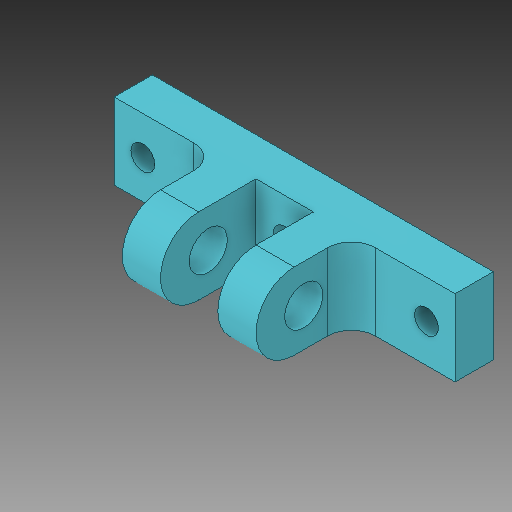
# Autodesk Inventor part: LowerSpringMountFront
Saved by Autodesk Inventor 2018.2 (Build 222227000, 227)
## iProperties
Created: 2018-03-25
Part Number: LowerSpringMountFront
Material: Generic
Document SubType Name: Modeling
Designer: MIABo
Density: 1 g/cm^3
Appearance: Default
Mass: 3.25903 g
Surface Area: 23.365 cm^2
Volume: 3.25903 cm^3
Author: MIABo
## iProperties of the stored document LowerSpringMountFront_3DPrint.ipt
Created: 2018-03-25
Part Number: LowerSpringMountFront_3DPrint
Material: Generic
Document SubType Name: Modeling
Designer: MIABo
Density: 1 g/cm^3
Appearance: Default
Author: MIABo
Autodesk Inventor part; units mm, degrees
ref_plane "YZ Plane" through (0, 0, 0) normal (1, 0, 0) x (0, 1, 0)
ref_plane "XZ Plane" through (0, 0, 0) normal (0, 1, 0) x (-1, 0, 0)
ref_plane "XY Plane" through (0, 0, 0) normal (0, 0, 1) x (1, 0, 0)
sketch "Sketch1" plane through (0, 0, 0) normal (0, 0, 1) x (1, 0, 0)
  line L0 (-22.6695, -5.08) -> (22.6695, -5.08)
  line L1 (22.6695, -5.08) -> (22.6695, 5.08)
  line L2 (22.6695, 5.08) -> (-22.6695, 5.08)
  line L3 (-22.6695, 5.08) -> (-22.6695, -5.08)
  line L4 (-22.6695, -5.08) -> (22.6695, 5.08) construction
  line L5 (22.6695, -5.08) -> (-22.6695, 5.08) construction
  point P0 (0, 0)
  dimension "d0" = 10.16
  dimension "d1" = 45.339
  constraints: 12 end point, 2 midpoint, 2 parallel, 1 horizontal, 1 perpendicular
  measures "d0" distance of L1.end L0.end
  measures "d1" distance of L1.end L2.end
extrude "Extrusion1" add sketch "Sketch1" along normal blind 5.08
sketch "Sketch2" plane through (0, 0, 0) normal (0, 0, -1) x (-1, 0, 0)
  line L0 (22.6695, 5.08) -> (22.6695, -5.08) projected
  line L1 (-22.6695, -5.08) -> (-22.6695, 5.08) projected
  line L2 (-22.6695, 5.08) -> (22.6695, 5.08) projected
  point P0 (0, 0)
  point P1 (18.8595, 0)
  point P2 (-18.8595, 0)
  dimension "d4" = 3.81
  dimension "d5" = 3.81
  dimension "d6" = 5.08
  dimension "d7" = 5.08
  measures "d4" distance from line of L0 point (18.86, 0)
  measures "d5" distance from line of L1 point (-18.86, 0)
  measures "d6" distance from line of L2 point (18.86, 0)
  measures "d7" distance from line of L2 point (-18.86, 0)
hole "Hole1" at (-18.8595, 0, 0) at (18.8595, 0, 0) direction (0, 0, 1) diameter 3.175 end through all
sketch "Sketch3" plane through (0, 0, 0) normal (0, 0, -1) x (-1, 0, 0)
  circle A0 centre (0, 0) radius 1.524
  dimension "d15" = 3.048
  constraints: 1 centre point, 1 coincident
  measures "d15" diameter of A0
extrude "Extrusion2" cut sketch "Sketch3" against normal through all
sketch "Sketch4" plane through (0, 0, 5.08) normal (0, 0, 1) x (1, 0, 0)
  line L0 (22.6695, 5.08) -> (-22.6695, 5.08) projected
  line L1 (-22.6695, -5.08) -> (22.6695, -5.08) projected
  line L2 (-3.81, 5.08) -> (-8.89, 5.08)
  line L3 (-8.89, 5.08) -> (-8.89, -5.08)
  line L4 (-8.89, -5.08) -> (-3.81, -5.08)
  line L5 (-3.81, -5.08) -> (-3.81, 5.08)
  line L6 (3.81, 5.08) -> (8.89, 5.08)
  line L7 (8.89, 5.08) -> (8.89, -5.08)
  line L8 (8.89, -5.08) -> (3.81, -5.08)
  line L9 (3.81, -5.08) -> (3.81, 5.08)
  point P0 (0, 0)
  dimension "d18" = 5.08
  dimension "d19" = 3.81
  dimension "d20" = 3.81
  dimension "d21" = 5.08
  constraints: 16 end point, 4 parallel, 4 point on line, 2 horizontal, 2 perpendicular
  measures "d18" distance between parallel lines of L5 L3
  measures "d19" distance from line of L5 point (0, 0)
  measures "d20" distance from line of L9 point (0, 0)
  measures "d21" distance between parallel lines of L9 L7
extrude "Extrusion3" add sketch "Sketch4" along normal blind 12.7 contours L7 L1 L9 L0 | L5 L1 L3 L0
sketch "Sketch5" plane through (-8.89, -5.08, 5.08) normal (-1, 0, 0) x (0, 0, 1)
  line L0 (12.7, 10.16) -> (12.7, 0) projected
  line L1 (0, 10.16) -> (12.7, 10.16) projected
  point P0 (-5.08, 5.08)
  point P1 (6.35, 5.08)
  dimension "d24" = 6.35
  dimension "d25" = 5.08
  measures "d24" distance from line of L0 point (6.35, 5.08)
  measures "d25" distance from line of L1 point (6.35, 5.08)
hole "Hole2" at (-8.89, 0, 11.43) direction (1, 0, 0) diameter 5.08 end through all
fillet "Fillet1" radius 3.175 2 edges at (-8.89, 0, 5.08) (8.89, 0, 5.08)
fillet "Fillet2" radius 5.08 4 edges at (6.35, -5.08, 17.78) (6.35, 5.08, 17.78) (-6.35, -5.08, 17.78) (-6.35, 5.08, 17.78)
body "Solid1"
